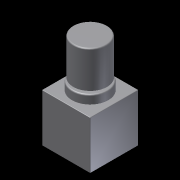
# Autodesk Inventor part: Taster
Saved by Autodesk Inventor 2011 SP1 (Build 150282100, 282)
## iProperties
Created: 2012-07-12
Part Number: Taster
Document SubType Name: Modeling
Designer: nfischer
Density: 1 g/cm^3
Author: nfischer
Autodesk Inventor part; units mm, degrees
ref_plane "YZ Plane" through (0, 0, 0) normal (1, 0, 0) x (0, 1, 0)
ref_plane "XZ Plane" through (0, 0, 0) normal (0, 1, 0) x (-1, 0, 0)
ref_plane "XY Plane" through (0, 0, 0) normal (0, 0, 1) x (1, 0, 0)
sketch "Skizze1" plane through (0, 0, 0) normal (0, 0, 1) x (1, 0, 0)
  line L0 (-5, 5) -> (5, 5)
  line L1 (5, 5) -> (5, -5)
  line L2 (5, -5) -> (-5, -5)
  line L3 (-5, -5) -> (-5, 5)
  point P0 (0, 0)
  point P1 (5, 0)
  point P2 (0, -5)
  dimension "d0" = 10
  dimension "d1" = 10
  constraints: 8 end point, 2 midpoint, 2 parallel, 1 horizontal, 1 horizontal alignment, 1 perpendicular, 1 vertical alignment
  measures "d0" distance of L2.end L0.start
  measures "d1" distance of L1.end L2.end
extrude "Extrusion1" add sketch "Skizze1" along normal blind 10
sketch "Skizze2" plane through (0, 0, 10) normal (0, 0, 1) x (1, 0, 0)
  circle A0 centre (0, 0) radius 3.75
  dimension "d4" = 7.5
  constraints: 1 centre point, 1 coincident
  measures "d4" diameter of A0
extrude "Extrusion2" add sketch "Skizze2" along normal blind 1.76
fillet "Rundung1" radius 0.25 1 edges at (-3.75, 0, 11.76)
sketch "Skizze3" plane through (0, 0, 11.76) normal (0, 0, 1) x (1, 0, 0)
  circle A0 centre (0, 0) radius 3.5 projected
  circle A1 centre (0, 0) radius 2.25
  dimension "d8" = 4.5
  constraints: 1 centre point, 1 coincident
  measures "d8" diameter of A1
extrude "Extrusion3" add sketch "Skizze3" along normal blind 0.5 contours A1
sketch "Skizze4" plane through (0, 0, 12.26) normal (0, 0, 1) x (1, 0, 0)
  circle A0 centre (0, 0) radius 2.25 projected
  circle A1 centre (0, 0) radius 3.5
  dimension "d11" = 7
  constraints: 1 centre point, 1 coincident
  measures "d11" diameter of A1
extrude "Extrusion4" add sketch "Skizze4" along normal blind 7.6 contours A0 | A1
fillet "Rundung2" radius 0.25 1 edges at (-3.5, 0, 19.86)
fillet "Rundung3" radius 0.1 12 edges at (-5, -5, 5) (-5, 5, 5) (-5, 0, 10) (0, -5, 10) (5, 0, 10) (5, -5, 5) (0, -5, 0) (-5, 0, 0) (0, 5, 0) (0, 5, 10) (5, 5, 5) (5, 0, 0)
sketch "Skizze5" plane through (-4.9, 5, 0.1) normal (0, 1, 0) x (1, 0, 0)
  point P0 (4.9, 0.1)
  point P1 (4.9, -1.1417)
hole "Hole2" at (0, 5, 1.2417) direction (0, -1, 0) diameter 2 depth 5 tip angle 118
